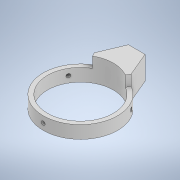
# Autodesk Inventor part: ring_light_holder
Saved by Autodesk Inventor 2021.2 (Build 252289000, 289)
## iProperties
Created: 2021-03-31
Part Number: ring_light_holder
Material: Generic
Document SubType Name: Modeling
Designer: yxion
Density: 1 g/cm^3
Appearance: Default
Author: yxion
Autodesk Inventor part; units mm, degrees
sketch "Sketch1" plane through (0, 0, 0) normal (0, 1, 0) x (-1, 0, 0)
  circle A0 centre (0, 0) radius 31
  circle A1 centre (0, 0) radius 35
  line L0 (17.3082, -30.4208) -> (7.8, -53)
  line L1 (7.8, -53) -> (-7.8, -53)
  line L2 (-7.8, -53) -> (-17.3082, -30.4208)
  line L3 (17.3082, -30.4208) -> (-15.7757, -30.4208) construction
  line L4 (-15.7757, -30.4208) -> (-17.7199, -30.4208) construction
  line L5 (0, 0) -> (0, -70.1965) construction
  dimension "d0" = 62
  dimension "d1" = 70
  dimension "d2" = 18
  dimension "d14" = 17.3082
  dimension "d15" = 17.3082
  dimension "d16" = 7.8
  dimension "d17" = 7.8
  constraints: 12 end point, 2 centre point, 2 coincident, 2 horizontal, 2 point on circle, 1 point on line, 1 vertical
  measures "d0" diameter of A0
  measures "d1" diameter of A1
  measures "d2" distance edge to line of A1 L1
  measures "d14" distance from line of L5 L0.start
  measures "d15" distance from line of L2.end L5
  measures "d16" distance from line of L5 L0.end
  measures "d17" distance from line of L1.end L5
extrude "Extrusion1" add sketch "Sketch1" along normal blind 12
sketch "Sketch2" plane through (7.8, 0, -53) normal (0, 0, -1) x (-1, 0, 0)
  line L0 (0, 0) -> (15.6, 0) projected
  line L1 (15.6, 0) -> (15.6, 12) projected
  line L2 (0, 12) -> (15.6, 12) projected
  line L3 (0, 0) -> (0, 12) projected
  circle A0 centre (7.8, 17) radius 2.6
  circle A1 centre (7.8, 5) radius 2.6
  line L4 (0, 12) -> (15.6, 12) construction
  line L5 (0, 0) -> (15.6, 0) construction
  line L6 (7.8, 17) -> (7.8, 22) construction
  line L7 (7.8, 10.4006) -> (15.6, 10.4006) construction
  line L8 (15.6, 0) -> (15.6, 12) construction
  line L9 (7.8, 8.8613) -> (0, 8.8613) construction
  line L10 (0, 0) -> (0, 12) construction
  line L11 (7.8, 17) -> (7.8, 1.4261) construction
  point P0 (7.8, 0)
  dimension "d5" = 5.2
  dimension "d6" = 5.2
  dimension "d7" = 12
  dimension "d11" = 5
  dimension "d20" = 5
  constraints: 8 end point, 2 centre point, 2 perpendicular, 2 point on line, 2 vertical, 1 parallel
  measures "d5" diameter of A0
  measures "d6" diameter of A1
  measures "d7" distance of L6.start A1.centre
  measures "d11" distance of L6.start L6.end
  measures "d20" distance from line of A1.centre L0
sketch "Sketch3" plane through (0, 12, 0) normal (0, 1, 0) x (1, 0, 0)
  line L0 (17.3082, 30.4208) -> (7.8, 53) projected
  line L1 (7.8, 53) -> (-7.8, 53) projected
  line L2 (-7.8, 53) -> (-17.3082, 30.4208) projected
  arc A0 (-17.3082, 30.4208) -> (17.3082, 30.4208) centre (0, 0) ccw projected
  circle A1 centre (0, 0) radius 31 projected
  arc A2 (-17.3082, 30.4208) -> (17.3082, 30.4208) centre (0, 0) ccw projected
  line L3 (17.3082, 30.4208) -> (15.4466, 26.8775)
  circle A3 centre (0, 0) radius 31 projected
  line L4 (-7.8, 53) -> (-17.3082, 30.4208) projected
  line L5 (-17.3082, 30.4208) -> (-15.4466, 26.8775)
  constraints: 4 end point, 4 other
extrude "Extrusion2" add sketch "Sketch3" along normal blind 10 contours L3 A1 L5 L2 L1 L0
extrude "Extrusion3" cut sketch "Sketch2" against normal blind 15 contours A0 | A1
ref_plane "Work Plane1" through (0, 0, 35) normal (0, 0, 1) x (1, 0, 0)
sketch "Sketch5" plane through (0, 0, 35) normal (0, 0, 1) x (1, 0, 0)
  line L0 (-17.3082, 0) -> (17.3082, 0) projected
  line L1 (17.3082, 0) -> (17.3082, 12) projected
  line L2 (-17.3082, 12) -> (17.3082, 12) projected
  line L3 (-17.3082, 0) -> (-17.3082, 12) projected
  line L4 (0, 0) -> (0, 4.5061) construction
  circle A0 centre (0, 6) radius 1.75
  dimension "d18" = 3.5
  dimension "d19" = 6
  constraints: 2 end point, 1 centre point, 1 point on line, 1 vertical
  measures "d18" diameter of A0
  measures "d19" distance from line of L0 A0.centre
extrude "Extrusion4" cut sketch "Sketch5" against normal blind 15 contours A0
ref_plane "Work Plane2" through (0, 0, 0) normal (0.866, 0, -0.5) x (0, 1, 0)
ref_plane "Work Plane3" through (30.3109, 0, -17.5) normal (0.866, 0, -0.5) x (0, 1, 0)
sketch "Sketch6" plane through (30.3109, 0, -17.5) normal (0.866, 0, -0.5) x (0, 1, 0)
  circle A0 centre (6, 0) radius 1.75
  line L0 (0, -17.6911) -> (0, 35) projected
  point P0 (0, 0)
  point P1 (0, -34.9993)
  dimension "d24" = 6
  dimension "d25" = 3.5
  constraints: 1 centre point
  measures "d24" distance from line of L0 A0.centre
  measures "d25" diameter of A0
extrude "Extrusion5" cut sketch "Sketch6" against normal blind 15
ref_plane "Work Plane6" through (-30.3109, 0, -17.5) normal (0.866, 0, 0.5) x (0, 1, 0)
ref_plane "Work Plane5" through (0, 0, 0) normal (0.866, 0, 0.5) x (0, 1, 0)
sketch "Sketch8" plane through (-30.3109, 0, -17.5) normal (0.866, 0, 0.5) x (0, 1, 0)
  circle A0 centre (6, 0) radius 1.75
  line L0 (0, -34.9993) -> (0, 35) projected
  point P0 (0, 0)
  point P1 (0, -17.6911)
  dimension "d33" = 3.5
  dimension "d34" = 6
  constraints: 1 centre point
  measures "d33" diameter of A0
  measures "d34" distance from line of L0 A0.centre
extrude "Extrusion7" cut sketch "Sketch8" along normal blind 15
body "Solid1"
